Autodesk Inventor part; units mm, degrees
(part 3 of 3)
  line L2025 (60.12, -86.945) -> (55.12, -86.945)
  line L2026 (55.12, -86.945) -> (55.12, -90.12)
  line L2027 (55.12, -90.12) -> (44.88, -90.12)
  line L2028 (44.88, -90.12) -> (44.88, -86.945)
  line L2029 (44.88, -86.945) -> (35.12, -86.945)
  line L2030 (35.12, -86.945) -> (35.12, -90.12)
  line L2031 (35.12, -90.12) -> (24.88, -90.12)
  line L2032 (24.88, -90.12) -> (24.88, -86.945)
  line L2033 (24.88, -86.945) -> (15.12, -86.945)
  line L2034 (15.12, -86.945) -> (15.12, -90.12)
  line L2035 (15.12, -90.12) -> (4.88, -90.12)
  line L2036 (4.88, -90.12) -> (4.88, -86.945)
  line L2037 (4.88, -86.945) -> (-4.88, -86.945)
  line L2038 (-4.88, -86.945) -> (-4.88, -90.12)
  line L2039 (-4.88, -90.12) -> (-15.12, -90.12)
  line L2040 (-15.12, -90.12) -> (-15.12, -86.945)
  line L2041 (-15.12, -86.945) -> (-24.88, -86.945)
  line L2042 (-24.88, -86.945) -> (-24.88, -90.12)
  line L2043 (-24.88, -90.12) -> (-35.12, -90.12)
  line L2044 (-35.12, -90.12) -> (-35.12, -86.945)
  line L2045 (-35.12, -86.945) -> (-44.88, -86.945)
  line L2046 (-44.88, -86.945) -> (-44.88, -90.12)
  line L2047 (-44.88, -90.12) -> (-55.12, -90.12)
  line L2048 (-55.12, -90.12) -> (-55.12, -86.945)
  line L2049 (-55.12, -86.945) -> (-60.12, -86.945)
  line L2050 (-60.12, -86.945) -> (-60.12, -74.88)
  line L2051 (-60.12, -74.88) -> (-56.945, -74.88)
  line L2052 (-56.945, -74.88) -> (-56.945, -65.12)
  line L2053 (-56.945, -65.12) -> (-60.12, -65.12)
  line L2054 (-60.12, -65.12) -> (-60.12, -54.88)
  line L2055 (-60.12, -54.88) -> (-56.945, -54.88)
  line L2056 (-56.945, -54.88) -> (-56.945, -45.12)
  line L2057 (-56.945, -45.12) -> (-60.12, -45.12)
  line L2058 (-60.12, -45.12) -> (-60.12, -34.88)
  line L2059 (-60.12, -34.88) -> (-56.945, -34.88)
  line L2060 (-56.945, -34.88) -> (-56.945, -25.12)
  line L2061 (-56.945, -25.12) -> (-60.12, -25.12)
  line L2062 (-60.12, -25.12) -> (-60.12, -14.88)
  line L2063 (-60.12, -14.88) -> (-56.945, -14.88)
  line L2064 (145.24, 90.12) -> (155.48, 90.12)
  line L2065 (155.48, 90.12) -> (155.48, 86.945)
  line L2066 (155.48, 86.945) -> (165.24, 86.945)
  line L2067 (165.24, 86.945) -> (165.24, 90.12)
  line L2068 (165.24, 90.12) -> (175.48, 90.12)
  line L2069 (175.48, 90.12) -> (175.48, 86.945)
  line L2070 (175.48, 86.945) -> (177.305, 86.945)
  line L2071 (177.305, 86.945) -> (177.305, 75.12)
  line L2072 (177.305, 75.12) -> (180.48, 75.12)
  line L2073 (180.48, 75.12) -> (180.48, 64.88)
  line L2074 (180.48, 64.88) -> (177.305, 64.88)
  line L2075 (177.305, 64.88) -> (177.305, 55.12)
  line L2076 (177.305, 55.12) -> (180.48, 55.12)
  line L2077 (180.48, 55.12) -> (180.48, 44.88)
  line L2078 (180.48, 44.88) -> (177.305, 44.88)
  line L2079 (177.305, 44.88) -> (177.305, 35.12)
  line L2080 (177.305, 35.12) -> (180.48, 35.12)
  line L2081 (180.48, 35.12) -> (180.48, 24.88)
  line L2082 (180.48, 24.88) -> (177.305, 24.88)
  line L2083 (177.305, 24.88) -> (177.305, 15.12)
  line L2084 (177.305, 15.12) -> (180.48, 15.12)
  line L2085 (180.48, 15.12) -> (180.48, 4.88)
  line L2086 (180.48, 4.88) -> (177.305, 4.88)
  line L2087 (177.305, 4.88) -> (177.305, -4.88)
  line L2088 (177.305, -4.88) -> (180.48, -4.88)
  line L2089 (180.48, -4.88) -> (180.48, -15.12)
  line L2090 (180.48, -15.12) -> (177.305, -15.12)
  line L2091 (177.305, -15.12) -> (177.305, -24.88)
  line L2092 (177.305, -24.88) -> (180.48, -24.88)
  line L2093 (180.48, -24.88) -> (180.48, -35.12)
  line L2094 (180.48, -35.12) -> (177.305, -35.12)
  line L2095 (177.305, -35.12) -> (177.305, -44.88)
  line L2096 (177.305, -44.88) -> (180.48, -44.88)
  line L2097 (180.48, -44.88) -> (180.48, -55.12)
  line L2098 (180.48, -55.12) -> (177.305, -55.12)
  line L2099 (177.305, -55.12) -> (177.305, -64.88)
  line L2100 (177.305, -64.88) -> (180.48, -64.88)
  line L2101 (180.48, -64.88) -> (180.48, -75.12)
  line L2102 (180.48, -75.12) -> (177.305, -75.12)
  line L2103 (177.305, -75.12) -> (177.305, -86.945)
  line L2104 (177.305, -86.945) -> (175.48, -86.945)
  line L2105 (175.48, -86.945) -> (175.48, -90.12)
  line L2106 (175.48, -90.12) -> (165.24, -90.12)
  line L2107 (165.24, -90.12) -> (165.24, -86.945)
  line L2108 (165.24, -86.945) -> (155.48, -86.945)
  line L2109 (155.48, -86.945) -> (155.48, -90.12)
  line L2110 (155.48, -90.12) -> (145.24, -90.12)
  line L2111 (145.24, -90.12) -> (145.24, -86.945)
  line L2112 (145.24, -86.945) -> (135.48, -86.945)
  line L2113 (135.48, -86.945) -> (135.48, -90.12)
  line L2114 (135.48, -90.12) -> (125.24, -90.12)
  line L2115 (125.24, -90.12) -> (125.24, -86.945)
  line L2116 (125.24, -86.945) -> (115.48, -86.945)
  line L2117 (115.48, -86.945) -> (115.48, -90.12)
  line L2118 (115.48, -90.12) -> (105.24, -90.12)
  line L2119 (105.24, -90.12) -> (105.24, -86.945)
  line L2120 (105.24, -86.945) -> (95.48, -86.945)
  line L2121 (95.48, -86.945) -> (95.48, -90.12)
  line L2122 (95.48, -90.12) -> (85.24, -90.12)
  line L2123 (85.24, -90.12) -> (85.24, -86.945)
  line L2124 (85.24, -86.945) -> (75.48, -86.945)
  line L2125 (75.48, -86.945) -> (75.48, -90.12)
  line L2126 (75.48, -90.12) -> (65.24, -90.12)
  line L2127 (65.24, -90.12) -> (65.24, -86.945)
  line L2128 (65.24, -86.945) -> (63.415, -86.945)
  line L2129 (63.415, -86.945) -> (63.415, -75.12)
  line L2130 (63.415, -75.12) -> (60.24, -75.12)
  line L2131 (60.24, -75.12) -> (60.24, -64.88)
  line L2132 (60.24, -64.88) -> (63.415, -64.88)
  line L2133 (63.415, -64.88) -> (63.415, -55.12)
  line L2134 (63.415, -55.12) -> (60.24, -55.12)
  line L2135 (60.24, -55.12) -> (60.24, -44.88)
  line L2136 (60.24, -44.88) -> (63.415, -44.88)
  line L2137 (63.415, -44.88) -> (63.415, -35.12)
  line L2138 (63.415, -35.12) -> (60.24, -35.12)
  line L2139 (60.24, -35.12) -> (60.24, -24.88)
  line L2140 (60.24, -24.88) -> (63.415, -24.88)
  line L2141 (63.415, -24.88) -> (63.415, -15.12)
  line L2142 (63.415, -15.12) -> (60.24, -15.12)
  line L2143 (60.24, -15.12) -> (60.24, -4.88)
  line L2144 (60.24, -4.88) -> (63.415, -4.88)
  line L2145 (63.415, -4.88) -> (63.415, 4.88)
  line L2146 (63.415, 4.88) -> (60.24, 4.88)
  line L2147 (60.24, 4.88) -> (60.24, 15.12)
  line L2148 (60.24, 15.12) -> (63.415, 15.12)
  line L2149 (63.415, 15.12) -> (63.415, 24.88)
  line L2150 (63.415, 24.88) -> (60.24, 24.88)
  line L2151 (60.24, 24.88) -> (60.24, 35.12)
  line L2152 (60.24, 35.12) -> (63.415, 35.12)
  line L2153 (63.415, 35.12) -> (63.415, 44.88)
  line L2154 (63.415, 44.88) -> (60.24, 44.88)
  line L2155 (60.24, 44.88) -> (60.24, 55.12)
  line L2156 (60.24, 55.12) -> (63.415, 55.12)
  line L2157 (63.415, 55.12) -> (63.415, 64.88)
  line L2158 (63.415, 64.88) -> (60.24, 64.88)
  line L2159 (60.24, 64.88) -> (60.24, 75.12)
  line L2160 (60.24, 75.12) -> (63.415, 75.12)
  line L2161 (63.415, 75.12) -> (63.415, 86.945)
  line L2162 (63.415, 86.945) -> (65.24, 86.945)
  line L2163 (65.24, 86.945) -> (65.24, 90.12)
  line L2164 (65.24, 90.12) -> (75.48, 90.12)
  line L2165 (75.48, 90.12) -> (75.48, 86.945)
  line L2166 (75.48, 86.945) -> (85.24, 86.945)
  line L2167 (85.24, 86.945) -> (85.24, 90.12)
  line L2168 (85.24, 90.12) -> (95.48, 90.12)
  line L2169 (95.48, 90.12) -> (95.48, 86.945)
  line L2170 (95.48, 86.945) -> (105.24, 86.945)
  line L2171 (105.24, 86.945) -> (105.24, 90.12)
  line L2172 (105.24, 90.12) -> (115.48, 90.12)
  line L2173 (115.48, 90.12) -> (115.48, 86.945)
  line L2174 (115.48, 86.945) -> (125.24, 86.945)
  line L2175 (125.24, 86.945) -> (125.24, 90.12)
  line L2176 (125.24, 90.12) -> (135.48, 90.12)
  line L2177 (135.48, 90.12) -> (135.48, 86.945)
  line L2178 (135.48, 86.945) -> (145.24, 86.945)
  line L2179 (145.24, 86.945) -> (145.24, 90.12)
  line L2180 (165.48, 14.88) -> (165.48, -14.88)
  line L2181 (165.48, -14.88) -> (175.24, -14.88)
  line L2182 (175.24, -14.88) -> (175.24, 14.88)
  line L2183 (175.24, 14.88) -> (165.48, 14.88)
  line L2184 (75.24, 14.88) -> (65.48, 14.88)
  line L2185 (65.48, 14.88) -> (65.48, -14.88)
  line L2186 (65.48, -14.88) -> (75.24, -14.88)
  line L2187 (75.24, -14.88) -> (75.24, 14.88)
  circle A54 centre (177.185, 50) radius 1.58
  circle A55 centre (177.185, -50) radius 1.58
  circle A56 centre (22.9972, 27.4451) radius 2.88
  line L2188 (43.695, -13.215) -> (40.125, -13.215)
  line L2189 (40.125, -13.215) -> (40.125, -2.025)
  line L2190 (40.125, -2.025) -> (43.695, -2.025)
  line L2191 (43.695, -2.025) -> (43.695, -13.215)
  circle A57 centre (45.72, 0) radius 0.958
  circle A58 centre (45.72, -15.24) radius 0.958
  circle A59 centre (38.1, -15.24) radius 0.958
  circle A60 centre (38.1, 0) radius 0.958
  circle A61 centre (22.9972, -27.4451) radius 2.88
  circle A62 centre (-15, 8.175) radius 11.12
  circle A63 centre (-22.9972, 54) radius 2.88
  circle A64 centre (-22.9972, -54) radius 2.88
  circle A65 centre (17.276, -59.1479) radius 0.958
  circle A66 centre (52.276, -59.1479) radius 0.958
  circle A67 centre (63.535, -50) radius 1.58
  circle A68 centre (63.535, 50) radius 1.58
  line L2192 (404.895, -13.335) -> (401.085, -13.335) projected
  line L2193 (401.085, -13.335) -> (401.085, -1.905) projected
  line L2194 (401.085, -1.905) -> (404.895, -1.905) projected
  line L2195 (404.895, -1.905) -> (404.895, -13.335) projected
  circle A69 centre (399.18, -15.24) radius 1.078 projected
  circle A70 centre (406.8, 0) radius 1.078 projected
  circle A71 centre (406.8, -15.24) radius 1.078 projected
  circle A72 centre (399.18, 0) radius 1.078 projected
  line L2196 (415.905, -48.5) -> (417.905, -48.5) projected
  line L2197 (417.905, -48.5) -> (417.905, -45) projected
  line L2198 (417.905, -45) -> (421.08, -45) projected
  line L2199 (421.08, -45) -> (421.08, -35) projected
  line L2200 (421.08, -35) -> (417.905, -35) projected
  line L2201 (417.905, -35) -> (417.905, -25) projected
  line L2202 (417.905, -25) -> (421.08, -25) projected
  line L2203 (421.08, -25) -> (421.08, -15) projected
  line L2204 (421.08, -15) -> (417.905, -15) projected
  line L2205 (417.905, -15) -> (417.905, -5) projected
  line L2206 (417.905, -5) -> (421.08, -5) projected
  line L2207 (421.08, -5) -> (421.08, 5) projected
  line L2208 (421.08, 5) -> (417.905, 5) projected
  line L2209 (417.905, 5) -> (417.905, 15) projected
  line L2210 (417.905, 15) -> (421.08, 15) projected
  line L2211 (421.08, 15) -> (421.08, 25) projected
  line L2212 (421.08, 25) -> (417.905, 25) projected
  line L2213 (417.905, 25) -> (417.905, 35) projected
  line L2214 (417.905, 35) -> (421.08, 35) projected
  line L2215 (421.08, 35) -> (421.08, 45) projected
  line L2216 (421.08, 45) -> (417.905, 45) projected
  line L2217 (417.905, 45) -> (417.905, 48.5) projected
  line L2218 (417.905, 48.5) -> (415.905, 48.5) projected
  line L2219 (415.905, 48.5) -> (415.905, 47.25) projected
  line L2220 (415.905, 47.25) -> (413.405, 47.25) projected
  line L2221 (413.405, 47.25) -> (413.405, 48.5) projected
  line L2222 (413.405, 48.5) -> (407.08, 48.5) projected
  line L2223 (407.08, 48.5) -> (407.08, 51.5) projected
  line L2224 (407.08, 51.5) -> (413.405, 51.5) projected
  line L2225 (413.405, 51.5) -> (413.405, 52.75) projected
  line L2226 (413.405, 52.75) -> (415.905, 52.75) projected
  line L2227 (415.905, 52.75) -> (415.905, 51.5) projected
  line L2228 (415.905, 51.5) -> (417.905, 51.5) projected
  line L2229 (417.905, 51.5) -> (417.905, 55) projected
  line L2230 (417.905, 55) -> (421.08, 55) projected
  line L2231 (421.08, 55) -> (421.08, 65) projected
  line L2232 (421.08, 65) -> (417.905, 65) projected
  line L2233 (417.905, 65) -> (417.905, 75) projected
  line L2234 (417.905, 75) -> (421.08, 75) projected
  line L2235 (421.08, 75) -> (421.08, 86.825) projected
  line L2236 (416.08, 86.825) -> (421.08, 86.825) projected
  line L2237 (416.08, 90) -> (416.08, 86.825) projected
  line L2238 (406.08, 90) -> (416.08, 90) projected
  line L2239 (406.08, 86.825) -> (406.08, 90) projected
  line L2240 (406.08, 86.825) -> (396.08, 86.825) projected
  line L2241 (396.08, 90) -> (396.08, 86.825) projected
  line L2242 (386.08, 90) -> (396.08, 90) projected
  line L2243 (386.08, 86.825) -> (386.08, 90) projected
  line L2244 (386.08, 86.825) -> (376.08, 86.825) projected
  line L2245 (376.08, 90) -> (376.08, 86.825) projected
  line L2246 (366.08, 90) -> (376.08, 90) projected
  line L2247 (366.08, 86.825) -> (366.08, 90) projected
  line L2248 (366.08, 86.825) -> (356.08, 86.825) projected
  line L2249 (356.08, 90) -> (356.08, 86.825) projected
  line L2250 (346.08, 90) -> (356.08, 90) projected
  line L2251 (346.08, 86.825) -> (346.08, 90) projected
  line L2252 (346.08, 86.825) -> (336.08, 86.825) projected
  line L2253 (336.08, 90) -> (336.08, 86.825) projected
  line L2254 (326.08, 90) -> (336.08, 90) projected
  line L2255 (326.08, 86.825) -> (326.08, 90) projected
  line L2256 (326.08, 86.825) -> (316.08, 86.825) projected
  line L2257 (316.08, 90) -> (316.08, 86.825) projected
  line L2258 (306.08, 90) -> (316.08, 90) projected
  line L2259 (306.08, 86.825) -> (306.08, 90) projected
  line L2260 (306.08, 86.825) -> (301.08, 86.825) projected
  line L2261 (301.08, 75) -> (301.08, 86.825) projected
  line L2262 (304.255, 75) -> (301.08, 75) projected
  line L2263 (304.255, 75) -> (304.255, 65) projected
  line L2264 (301.08, 65) -> (304.255, 65) projected
  line L2265 (301.08, 55) -> (301.08, 65) projected
  line L2266 (304.255, 55) -> (301.08, 55) projected
  line L2267 (304.255, 55) -> (304.255, 45) projected
  line L2268 (301.08, 45) -> (304.255, 45) projected
  line L2269 (301.08, 35) -> (301.08, 45) projected
  line L2270 (304.255, 35) -> (301.08, 35) projected
  line L2271 (304.255, 35) -> (304.255, 25) projected
  line L2272 (301.08, 25) -> (304.255, 25) projected
  line L2273 (301.08, 15) -> (301.08, 25) projected
  line L2274 (304.255, 15) -> (301.08, 15) projected
  line L2275 (304.255, 15) -> (304.255, 5) projected
  line L2276 (301.08, 5) -> (304.255, 5) projected
  line L2277 (301.08, -5) -> (301.08, 5) projected
  line L2278 (304.255, -5) -> (301.08, -5) projected
  line L2279 (304.255, -5) -> (304.255, -15) projected
  line L2280 (301.08, -15) -> (304.255, -15) projected
  line L2281 (301.08, -25) -> (301.08, -15) projected
  line L2282 (304.255, -25) -> (301.08, -25) projected
  line L2283 (304.255, -25) -> (304.255, -35) projected
  line L2284 (301.08, -35) -> (304.255, -35) projected
  line L2285 (301.08, -45) -> (301.08, -35) projected
  line L2286 (304.255, -45) -> (301.08, -45) projected
  line L2287 (304.255, -45) -> (304.255, -55) projected
  line L2288 (301.08, -55) -> (304.255, -55) projected
  line L2289 (301.08, -65) -> (301.08, -55) projected
  line L2290 (304.255, -65) -> (301.08, -65) projected
  line L2291 (304.255, -65) -> (304.255, -75) projected
  line L2292 (301.08, -75) -> (304.255, -75) projected
  line L2293 (301.08, -75) -> (301.08, -86.825) projected
  line L2294 (301.08, -86.825) -> (306.08, -86.825) projected
  line L2295 (306.08, -86.825) -> (306.08, -90) projected
  line L2296 (306.08, -90) -> (316.08, -90) projected
  line L2297 (316.08, -90) -> (316.08, -86.825) projected
  line L2298 (316.08, -86.825) -> (326.08, -86.825) projected
  line L2299 (326.08, -86.825) -> (326.08, -90) projected
  line L2300 (326.08, -90) -> (336.08, -90) projected
  line L2301 (336.08, -90) -> (336.08, -86.825) projected
  line L2302 (336.08, -86.825) -> (346.08, -86.825) projected
  line L2303 (346.08, -86.825) -> (346.08, -90) projected
  line L2304 (346.08, -90) -> (356.08, -90) projected
  line L2305 (356.08, -90) -> (356.08, -86.825) projected
  line L2306 (356.08, -86.825) -> (366.08, -86.825) projected
  line L2307 (366.08, -86.825) -> (366.08, -90) projected
  line L2308 (366.08, -90) -> (376.08, -90) projected
  line L2309 (376.08, -90) -> (376.08, -86.825) projected
  line L2310 (376.08, -86.825) -> (386.08, -86.825) projected
  line L2311 (386.08, -86.825) -> (386.08, -90) projected
  line L2312 (386.08, -90) -> (396.08, -90) projected
  line L2313 (396.08, -90) -> (396.08, -86.825) projected
  line L2314 (396.08, -86.825) -> (406.08, -86.825) projected
  line L2315 (406.08, -86.825) -> (406.08, -90) projected
  line L2316 (406.08, -90) -> (416.08, -90) projected
  line L2317 (416.08, -90) -> (416.08, -86.825) projected
  line L2318 (416.08, -86.825) -> (421.08, -86.825) projected
  line L2319 (421.08, -86.825) -> (421.08, -75) projected
  line L2320 (421.08, -75) -> (417.905, -75) projected
  line L2321 (417.905, -75) -> (417.905, -65) projected
  line L2322 (417.905, -65) -> (421.08, -65) projected
  line L2323 (421.08, -65) -> (421.08, -55) projected
  line L2324 (421.08, -55) -> (417.905, -55) projected
  line L2325 (417.905, -55) -> (417.905, -51.5) projected
  line L2326 (417.905, -51.5) -> (415.905, -51.5) projected
  line L2327 (415.905, -51.5) -> (415.905, -52.75) projected
  line L2328 (415.905, -52.75) -> (413.405, -52.75) projected
  line L2329 (413.405, -52.75) -> (413.405, -51.5) projected
  line L2330 (413.405, -51.5) -> (407.08, -51.5) projected
  line L2331 (407.08, -51.5) -> (407.08, -48.5) projected
  line L2332 (407.08, -48.5) -> (413.405, -48.5) projected
  line L2333 (413.405, -48.5) -> (413.405, -47.25) projected
  line L2334 (413.405, -47.25) -> (415.905, -47.25) projected
  line L2335 (415.905, -47.25) -> (415.905, -48.5) projected
  circle A73 centre (384.0772, -27.4451) radius 3 projected
  circle A74 centre (338.0828, 54) radius 3 projected
  circle A75 centre (384.0772, 27.4451) radius 3 projected
  circle A76 centre (338.0828, -54) radius 3 projected
  circle A77 centre (346.08, 8.175) radius 11 projected
  point P0 (0, 0)
  dimension "d0" = 0.12
  dimension "d1" = 0.12
  dimension "d2" = 0.12
  dimension "d3" = 0.12
  dimension "d4" = 0.12
  dimension "d5" = 0.12
  dimension "d6" = 0.12
  dimension "d7" = 0.12
  dimension "d8" = 0.12
  dimension "d9" = 0.12
  dimension "d10" = 0.12
  dimension "d11" = 0.12
  dimension "d12" = 0.12
  dimension "d13" = 0.12
  dimension "d14" = 0.12
  dimension "d15" = 0.12
  dimension "d16" = 0.12
  dimension "d17" = 0.12
  dimension "d18" = 0.12
  dimension "d19" = 0.12
  dimension "d20" = 0.12
  dimension "d21" = 0.12
  dimension "d22" = 0.12
  dimension "d23" = 0.12
  dimension "d24" = 0.12
  dimension "d25" = 0.12
  dimension "d26" = 0.12
  dimension "d27" = 0.12
  dimension "d28" = 0.12
  dimension "d29" = 0.12
  dimension "d30" = 0.12
  dimension "d31" = 0.12
  dimension "d32" = 0.12
  dimension "d33" = 0.12
  dimension "d34" = 0.12
  dimension "d35" = 0.12
  dimension "d36" = 0.12
  dimension "d37" = 0.12
  dimension "d38" = 0.12
  constraints: 1904 end point, 25 centre point, 938 other
  measures "d0" distance between parallel lines of L995 L1096
  measures "d1" radial gap between concentric circles of A27 A35
  measures "d2" radial gap between concentric circles of A29 A36
  measures "d3" distance between parallel lines of L955 L1239
  measures "d4" radial gap between concentric circles of A28 A37
  measures "d5" radial gap between concentric circles of A26 A38
  measures "d6" radial gap between concentric circles of A32 A39
  measures "d7" radial gap between concentric circles of A30 A40
  measures "d8" radial gap between concentric circles of A24 A41
  measures "d9" radial gap between concentric circles of A25 A42
  measures "d10" radial gap between concentric circles of A31 A43
  measures "d11" radial gap between concentric circles of A34 A44
  measures "d12" distance between parallel lines of L685 L1384
  measures "d13" distance between parallel lines of L575 L1388
  measures "d14" distance between parallel lines of L876 L1504
  measures "d15" distance between parallel lines of L948 L1620
  measures "d16" distance between parallel lines of L567 L1723
  measures "d17" distance between parallel lines of L337 L1724
  measures "d18" distance between parallel lines of L233 L1824
  measures "d19" distance between parallel lines of L87 L1924
  measures "d20" distance between parallel lines of L359 L2064
  measures "d21" distance between parallel lines of L344 L2180
  measures "d22" distance between parallel lines of L349 L2184
  measures "d23" radial gap between concentric circles of A12 A54
  measures "d24" radial gap between concentric circles of A11 A55
  measures "d25" radial gap between concentric circles of A8 A56
  measures "d26" distance between parallel lines of L3 L2191
  measures "d27" radial gap between concentric circles of A3 A57
  measures "d28" radial gap between concentric circles of A4 A58
  measures "d29" radial gap between concentric circles of A2 A59
  measures "d30" radial gap between concentric circles of A5 A60
  measures "d31" radial gap between concentric circles of A6 A61
  measures "d32" radial gap between concentric circles of A10 A62
  measures "d33" radial gap between concentric circles of A7 A63
  measures "d34" radial gap between concentric circles of A9 A64
  measures "d35" radial gap between concentric circles of A1 A65
  measures "d36" radial gap between concentric circles of A0 A66
  measures "d37" radial gap between concentric circles of A13 A67
  measures "d38" radial gap between concentric circles of A14 A68
extrude "Extrusion1" add sketch "Sketch1" along normal blind 3.175 contours A0 | A1 | L0 L1 L2 L3 | A2 | A3 | A4 | A5 | L143 L142 L141 L140 L139 L138 L137 L136 L135 L134 L133 L132 L131 L130 L129 L128 L127 L126 L125 L124 L123 L122 L121 L120 L119 L118 L117 L116 L115 L114 L113 L112 L111 L110 L109 L108 L107 L106 L105 L104 L103 L102 L101 L100 L99 L98 L97 L96 L95 L94 L93 L92 L91 L90 L89 L88 L87 L86 L85 L84 L83 L82 L81 L80 L79 L78 L77 L76 L75 L74 L73 L72 L71 L70 L69 L68 L67 L66 L65 L64 L63 L62 L61 L60 L59 L58 L57 L56 L55 L54 L53 L52 L51 L50 L49 L48 L47 L46 L45 L44 L43 L42 L41 L40 L39 L38 L37 L36 L35 L34 L33 L32 L31 L30 L29 L28 L27 L26 L25 L24 L23 L22 L21 L20 L19 L18 L17 L16 L15 L14 L13 L12 L11 L10 L9 L8 L7 L6 L5 L4 | A6 | A7 | A8 | A9 | L243 L242 L241 L240 L239 L238 L237 L236 L235 L234 L233 L232 L231 L230 L229 L228 L227 L226 L225 L224 L223 L222 L221 L220 L219 L218 L217 L216 L215 L214 L213 L212 L211 L210 L209 L208 L207 L206 L205 L204 L203 L202 L201 L200 L199 L198 L197 L196 L195 L194 L193 L192 L191 L190 L189 L188 L187 L186 L185 L184 L183 L182 L181 L180 L179 L178 L177 L176 L175 L174 L173 L172 L171 L170 L169 L168 L167 L166 L165 L164 L163 L162 L161 L160 L159 L158 L157 L156 L155 L154 L153 L152 L151 L150 L149 L148 L147 L146 L145 L144 | L343 L342 L341 L340 L339 L338 L337 L336 L335 L334 L333 L332 L331 L330 L329 L328 L327 L326 L325 L324 L323 L322 L321 L320 L319 L318 L317 L316 L315 L314 L313 L312 L311 L310 L309 L308 L307 L306 L305 L304 L303 L302 L301 L300 L299 L298 L297 L296 L295 L294 L293 L292 L291 L290 L289 L288 L287 L286 L285 L284 L283 L282 L281 L280 L279 L278 L277 L276 L275 L274 L273 L272 L271 L270 L269 L268 L267 L266 L265 L264 L263 L262 L261 L260 L259 L258 L257 L256 L255 L254 L253 L252 L251 L250 L249 L248 L247 L246 L245 L244 | L344 L345 L346 L347 | L348 L349 L350 L351 | A11 | A12 | A13 | A14 | L467 L466 L465 L464 L463 L462 L461 L460 L459 L458 L457 L456 L455 L454 L453 L452 L451 L450 L449 L448 L447 L446 L445 L444 L443 L442 L441 L440 L439 L438 L437 L436 L435 L434 L433 L432 L431 L430 L429 L428 L427 L426 L425 L424 L423 L422 L421 L420 L419 L418 L417 L416 L415 L414 L413 L412 L411 L410 L409 L408 L407 L406 L405 L404 L403 L402 L401 L400 L399 L398 L397 L396 L395 L394 L393 L392 L391 L390 L389 L388 L387 L386 L385 L384 L383 L382 L381 L380 L379 L378 L377 L376 L375 L374 L373 L372 L371 L370 L369 L368 L367 L366 L365 L364 L363 L362 L361 L360 L359 L358 L357 L356 L355 L354 L353 L352 | L567 L566 L565 L564 L563 L562 L561 L560 L559 L558 L557 L556 L555 L554 L553 L552 L551 L550 L549 L548 L547 L546 L545 L544 L543 L542 L541 L540 L539 L538 L537 L536 L535 L534 L533 L532 L531 L530 L529 L528 L527 L526 L525 L524 L523 L522 L521 L520 L519 L518 L517 L516 L515 L514 L513 L512 L511 L510 L509 L508 L507 L506 L505 L504 L503 L502 L501 L500 L499 L498 L497 L496 L495 L494 L493 L492 L491 L490 L489 L488 L487 L486 L485 L484 L483 L482 L481 L480 L479 L478 L477 L476 L475 L474 L473 L472 L471 L470 L469 L468 | L683 L682 L681 L680 L679 L678 L677 L676 L675 L674 L673 L672 L671 L670 L669 L668 L667 L666 L665 L664 L663 L662 L661 L660 L659 L658 L657 L656 L655 L654 L653 L652 L651 L650 L649 L648 L647 L646 L645 L644 L643 L642 L641 L640 L639 L638 L637 L636 L635 L634 L633 L632 L631 L630 L629 L628 L627 L626 L625 L624 L623 L622 L621 L620 L619 L618 L617 L616 L615 L614 L613 L612 L611 L610 L609 L608 L607 L606 L605 L604 L603 L602 L601 L600 L599 L598 L597 L596 L595 L594 L593 L592 L591 L590 L589 L588 L587 L586 L585 L584 L583 L582 L581 L580 L579 L578 L577 L576 L575 L574 L573 L572 L571 L570 L569 L568 | L684 L685 L686 L687 | L947 L946 L945 L944 L943 L942 L941 L940 L939 L938 L937 L936 L935 L934 L933 L932 L931 L930 L929 L928 L927 L926 L925 L924 L923 L922 L921 L920 L919 L918 L917 L916 L915 L914 L913 L912 L911 L910 L909 L908 L907 L906 L905 L904 L903 L902 L901 L900 L899 L898 L897 L896 L895 L894 L893 L892 L891 L890 L889 L888 L887 L886 L885 L884 L883 L882 L881 L880 L879 L878 L877 L876 L875 L874 L873 L872 L871 L870 L869 L868 L867 L866 L865 L864 L863 L862 L861 L860 L859 L858 L857 L856 L855 L854 L853 L852 L851 L850 L849 L848 L847 L846 L845 L844 L843 L842 L841 L840 L839 L838 L837 L836 L835 L834 L833 L832 | L948 L949 L950 L951 | A24 | A25 | L952 L953 L954 L955 | A27 | A28 | A29 | L1095 L1094 L1093 L1092 L1091 L1090 L1089 L1088 L1087 L1086 L1085 L1084 L1083 L1082 L1081 L1080 L1079 L1078 L1077 L1076 L1075 L1074 L1073 L1072 L1071 L1070 L1069 L1068 L1067 L1066 L1065 L1064 L1063 L1062 L1061 L1060 L1059 L1058 L1057 L1056 L1055 L1054 L1053 L1052 L1051 L1050 L1049 L1048 L1047 L1046 L1045 L1044 L1043 L1042 L1041 L1040 L1039 L1038 L1037 L1036 L1035 L1034 L1033 L1032 L1031 L1030 L1029 L1028 L1027 L1026 L1025 L1024 L1023 L1022 L1021 L1020 L1019 L1018 L1017 L1016 L1015 L1014 L1013 L1012 L1011 L1010 L1009 L1008 L1007 L1006 L1005 L1004 L1003 L1002 L1001 L1000 L999 L998 L997 L996 L995 L994 L993 L992 L991 L990 L989 L988 L987 L986 L985 L984 L983 L982 L981 L980 L979 L978 L977 L976 L975 L974 L973 L972 L971 L970 L969 L968 L967 L966 L965 L964 L963 L962 L961 L960 L959 L958 L957 L956 | A30 | A31 | A32 | A34 | L1096 L1097 L1098 L1099 L1100 L1101 L1102 L1103 L1104 L1105 L1106 L1107 L1108 L1109 L1110 L1111 L1112 L1113 L1114 L1115 L1116 L1117 L1118 L1119 L1120 L1121 L1122 L1123 L1124 L1125 L1126 L1127 L1128 L1129 L1130 L1131 L1132 L1133 L1134 L1135 L1136 L1137 L1138 L1139 L1140 L1141 L1142 L1143 L1144 L1145 L1146 L1147 L1148 L1149 L1150 L1151 L1152 L1153 L1154 L1155 L1156 L1157 L1158 L1159 L1160 L1161 L1162 L1163 L1164 L1165 L1166 L1167 L1168 L1169 L1170 L1171 L1172 L1173 L1174 L1175 L1176 L1177 L1178 L1179 L1180 L1181 L1182 L1183 L1184 L1185 L1186 L1187 L1188 L1189 L1190 L1191 L1192 L1193 L1194 L1195 L1196 L1197 L1198 L1199 L1200 L1201 L1202 L1203 L1204 L1205 L1206 L1207 L1208 L1209 L1210 L1211 L1212 L1213 L1214 L1215 L1216 L1217 L1218 L1219 L1220 L1221 L1222 L1223 L1224 L1225 L1226 L1227 L1228 L1229 L1230 L1231 L1232 L1233 L1234 L1235 | A38 | L1388 L1389 L1390 L1391 L1392 L1393 L1394 L1395 L1396 L1397 L1398 L1399 L1400 L1401 L1402 L1403 L1404 L1405 L1406 L1407 L1408 L1409 L1410 L1411 L1412 L1413 L1414 L1415 L1416 L1417 L1418 L1419 L1420 L1421 L1422 L1423 L1424 L1425 L1426 L1427 L1428 L1429 L1430 L1431 L1432 L1433 L1434 L1435 L1436 L1437 L1438 L1439 L1440 L1441 L1442 L1443 L1444 L1445 L1446 L1447 L1448 L1449 L1450 L1451 L1452 L1453 L1454 L1455 L1456 L1457 L1458 L1459 L1460 L1461 L1462 L1463 L1464 L1465 L1466 L1467 L1468 L1469 L1470 L1471 L1472 L1473 L1474 L1475 L1476 L1477 L1478 L1479 L1480 L1481 L1482 L1483 L1484 L1485 L1486 L1487 L1488 L1489 L1490 L1491 L1492 L1493 L1494 L1495 L1496 L1497 L1498 L1499 L1500 L1501 L1502 L1503 | L1504 L1505 L1506 L1507 L1508 L1509 L1510 L1511 L1512 L1513 L1514 L1515 L1516 L1517 L1518 L1519 L1520 L1521 L1522 L1523 L1524 L1525 L1526 L1527 L1528 L1529 L1530 L1531 L1532 L1533 L1534 L1535 L1536 L1537 L1538 L1539 L1540 L1541 L1542 L1543 L1544 L1545 L1546 L1547 L1548 L1549 L1550 L1551 L1552 L1553 L1554 L1555 L1556 L1557 L1558 L1559 L1560 L1561 L1562 L1563 L1564 L1565 L1566 L1567 L1568 L1569 L1570 L1571 L1572 L1573 L1574 L1575 L1576 L1577 L1578 L1579 L1580 L1581 L1582 L1583 L1584 L1585 L1586 L1587 L1588 L1589 L1590 L1591 L1592 L1593 L1594 L1595 L1596 L1597 L1598 L1599 L1600 L1601 L1602 L1603 L1604 L1605 L1606 L1607 L1608 L1609 L1610 L1611 L1612 L1613 L1614 L1615 L1616 L1617 L1618 L1619 | L1723 L1722 L1721 L1720 L1719 L1718 L1717 L1716 L1715 L1714 L1713 L1712 L1711 L1710 L1709 L1708 L1707 L1706 L1705 L1704 L1703 L1702 L1701 L1700 L1699 L1698 L1697 L1696 L1695 L1694 L1693 L1692 L1691 L1690 L1689 L1688 L1687 L1686 L1685 L1684 L1683 L1682 L1681 L1680 L1679 L1678 L1677 L1676 L1675 L1674 L1673 L1672 L1671 L1670 L1669 L1668 L1667 L1666 L1665 L1664 L1663 L1662 L1661 L1660 L1659 L1658 L1657 L1656 L1655 L1654 L1653 L1652 L1651 L1650 L1649 L1648 L1647 L1646 L1645 L1644 L1643 L1642 L1641 L1640 L1639 L1638 L1637 L1636 L1635 L1634 L1633 L1632 L1631 L1630 L1629 L1628 L1627 L1626 L1625 L1624 | L1724 L1725 L1726 L1727 L1728 L1729 L1730 L1731 L1732 L1733 L1734 L1735 L1736 L1737 L1738 L1739 L1740 L1741 L1742 L1743 L1744 L1745 L1746 L1747 L1748 L1749 L1750 L1751 L1752 L1753 L1754 L1755 L1756 L1757 L1758 L1759 L1760 L1761 L1762 L1763 L1764 L1765 L1766 L1767 L1768 L1769 L1770 L1771 L1772 L1773 L1774 L1775 L1776 L1777 L1778 L1779 L1780 L1781 L1782 L1783 L1784 L1785 L1786 L1787 L1788 L1789 L1790 L1791 L1792 L1793 L1794 L1795 L1796 L1797 L1798 L1799 L1800 L1801 L1802 L1803 L1804 L1805 L1806 L1807 L1808 L1809 L1810 L1811 L1812 L1813 L1814 L1815 L1816 L1817 L1818 L1819 L1820 L1821 L1822 L1823 | L1824 L1825 L1826 L1827 L1828 L1829 L1830 L1831 L1832 L1833 L1834 L1835 L1836 L1837 L1838 L1839 L1840 L1841 L1842 L1843 L1844 L1845 L1846 L1847 L1848 L1849 L1850 L1851 L1852 L1853 L1854 L1855 L1856 L1857 L1858 L1859 L1860 L1861 L1862 L1863 L1864 L1865 L1866 L1867 L1868 L1869 L1870 L1871 L1872 L1873 L1874 L1875 L1876 L1877 L1878 L1879 L1880 L1881 L1882 L1883 L1884 L1885 L1886 L1887 L1888 L1889 L1890 L1891 L1892 L1893 L1894 L1895 L1896 L1897 L1898 L1899 L1900 L1901 L1902 L1903 L1904 L1905 L1906 L1907 L1908 L1909 L1910 L1911 L1912 L1913 L1914 L1915 L1916 L1917 L1918 L1919 L1920 L1921 L1922 L1923 | L1924 L1925 L1926 L1927 L1928 L1929 L1930 L1931 L1932 L1933 L1934 L1935 L1936 L1937 L1938 L1939 L1940 L1941 L1942 L1943 L1944 L1945 L1946 L1947 L1948 L1949 L1950 L1951 L1952 L1953 L1954 L1955 L1956 L1957 L1958 L1959 L1960 L1961 L1962 L1963 L1964 L1965 L1966 L1967 L1968 L1969 L1970 L1971 L1972 L1973 L1974 L1975 L1976 L1977 L1978 L1979 L1980 L1981 L1982 L1983 L1984 L1985 L1986 L1987 L1988 L1989 L1990 L1991 L1992 L1993 L1994 L1995 L1996 L1997 L1998 L1999 L2000 L2001 L2002 L2003 L2004 L2005 L2006 L2007 L2008 L2009 L2010 L2011 L2012 L2013 L2014 L2015 L2016 L2017 L2018 L2019 L2020 L2021 L2022 L2023 L2024 L2025 L2026 L2027 L2028 L2029 L2030 L2031 L2032 L2033 L2034 L2035 L2036 L2037 L2038 L2039 L2040 L2041 L2042 L2043 L2044 L2045 L2046 L2047 L2048 L2049 L2050 L2051 L2052 L2053 L2054 L2055 L2056 L2057 L2058 L2059 L2060 L2061 L2062 L2063 | L2064 L2065 L2066 L2067 L2068 L2069 L2070 L2071 L2072 L2073 L2074 L2075 L2076 L2077 L2078 L2079 L2080 L2081 L2082 L2083 L2084 L2085 L2086 L2087 L2088 L2089 L2090 L2091 L2092 L2093 L2094 L2095 L2096 L2097 L2098 L2099 L2100 L2101 L2102 L2103 L2104 L2105 L2106 L2107 L2108 L2109 L2110 L2111 L2112 L2113 L2114 L2115 L2116 L2117 L2118 L2119 L2120 L2121 L2122 L2123 L2124 L2125 L2126 L2127 L2128 L2129 L2130 L2131 L2132 L2133 L2134 L2135 L2136 L2137 L2138 L2139 L2140 L2141 L2142 L2143 L2144 L2145 L2146 L2147 L2148 L2149 L2150 L2151 L2152 L2153 L2154 L2155 L2156 L2157 L2158 L2159 L2160 L2161 L2162 L2163 L2164 L2165 L2166 L2167 L2168 L2169 L2170 L2171 L2172 L2173 L2174 L2175 L2176 L2177 L2178 L2179 | A62
ref_plane "Work Plane2" through (361.08, 0, 0) normal (0, 0, 1) x (1, 0, 0)
sketch "Sketch3" plane through (361.08, 0, 0) normal (0, 0, 1) x (1, 0, 0)
  line L0 (43.815, -13.335) -> (40.005, -13.335) projected
  line L1 (40.005, -13.335) -> (40.005, -1.905) projected
  line L2 (40.005, -1.905) -> (43.815, -1.905) projected
  line L3 (43.815, -1.905) -> (43.815, -13.335) projected
  circle A0 centre (38.1, -15.24) radius 1.078 projected
  circle A1 centre (45.72, 0) radius 1.078 projected
  circle A2 centre (45.72, -15.24) radius 1.078 projected
  circle A3 centre (38.1, 0) radius 1.078 projected
  line L4 (54.825, -48.5) -> (56.825, -48.5) projected
  line L5 (56.825, -48.5) -> (56.825, -45) projected
  line L6 (56.825, -45) -> (60, -45) projected
  line L7 (60, -45) -> (60, -35) projected
  line L8 (60, -35) -> (56.825, -35) projected
  line L9 (56.825, -35) -> (56.825, -25) projected
  line L10 (56.825, -25) -> (60, -25) projected
  line L11 (60, -25) -> (60, -15) projected
  line L12 (60, -15) -> (56.825, -15) projected
  line L13 (56.825, -15) -> (56.825, -5) projected
  line L14 (56.825, -5) -> (60, -5) projected
  line L15 (60, -5) -> (60, 5) projected
  line L16 (60, 5) -> (56.825, 5) projected
  line L17 (56.825, 5) -> (56.825, 15) projected
  line L18 (56.825, 15) -> (60, 15) projected
  line L19 (60, 15) -> (60, 25) projected
  line L20 (60, 25) -> (56.825, 25) projected
  line L21 (56.825, 25) -> (56.825, 35) projected
  line L22 (56.825, 35) -> (60, 35) projected
  line L23 (60, 35) -> (60, 45) projected
  line L24 (60, 45) -> (56.825, 45) projected
  line L25 (56.825, 45) -> (56.825, 48.5) projected
  line L26 (56.825, 48.5) -> (54.825, 48.5) projected
  line L27 (54.825, 48.5) -> (54.825, 47.25) projected
  line L28 (54.825, 47.25) -> (52.325, 47.25) projected
  line L29 (52.325, 47.25) -> (52.325, 48.5) projected
  line L30 (52.325, 48.5) -> (46, 48.5) projected
  line L31 (46, 48.5) -> (46, 51.5) projected
  line L32 (46, 51.5) -> (52.325, 51.5) projected
  line L33 (52.325, 51.5) -> (52.325, 52.75) projected
  line L34 (52.325, 52.75) -> (54.825, 52.75) projected
  line L35 (54.825, 52.75) -> (54.825, 51.5) projected
  line L36 (54.825, 51.5) -> (56.825, 51.5) projected
  line L37 (56.825, 51.5) -> (56.825, 55) projected
  line L38 (56.825, 55) -> (60, 55) projected
  line L39 (60, 55) -> (60, 65) projected
  line L40 (60, 65) -> (56.825, 65) projected
  line L41 (56.825, 65) -> (56.825, 75) projected
  line L42 (56.825, 75) -> (60, 75) projected
  line L43 (60, 75) -> (60, 86.825) projected
  line L44 (55, 86.825) -> (60, 86.825) projected
  line L45 (55, 90) -> (55, 86.825) projected
  line L46 (45, 90) -> (55, 90) projected
  line L47 (45, 86.825) -> (45, 90) projected
  line L48 (45, 86.825) -> (35, 86.825) projected
  line L49 (35, 90) -> (35, 86.825) projected
  line L50 (25, 90) -> (35, 90) projected
  line L51 (25, 86.825) -> (25, 90) projected
  line L52 (25, 86.825) -> (15, 86.825) projected
  line L53 (15, 90) -> (15, 86.825) projected
  line L54 (5, 90) -> (15, 90) projected
  line L55 (5, 86.825) -> (5, 90) projected
  line L56 (5, 86.825) -> (-5, 86.825) projected
  line L57 (-5, 90) -> (-5, 86.825) projected
  line L58 (-15, 90) -> (-5, 90) projected
  line L59 (-15, 86.825) -> (-15, 90) projected
  line L60 (-15, 86.825) -> (-25, 86.825) projected
  line L61 (-25, 90) -> (-25, 86.825) projected
  line L62 (-35, 90) -> (-25, 90) projected
  line L63 (-35, 86.825) -> (-35, 90) projected
  line L64 (-35, 86.825) -> (-45, 86.825) projected
  line L65 (-45, 90) -> (-45, 86.825) projected
  line L66 (-55, 90) -> (-45, 90) projected
  line L67 (-55, 86.825) -> (-55, 90) projected
  line L68 (-55, 86.825) -> (-60, 86.825) projected
  line L69 (-60, 75) -> (-60, 86.825) projected
  line L70 (-56.825, 75) -> (-60, 75) projected
  line L71 (-56.825, 75) -> (-56.825, 65) projected
  line L72 (-60, 65) -> (-56.825, 65) projected
  line L73 (-60, 55) -> (-60, 65) projected
  line L74 (-56.825, 55) -> (-60, 55) projected
  line L75 (-56.825, 55) -> (-56.825, 45) projected
  line L76 (-60, 45) -> (-56.825, 45) projected
  line L77 (-60, 35) -> (-60, 45) projected
  line L78 (-56.825, 35) -> (-60, 35) projected
  line L79 (-56.825, 35) -> (-56.825, 25) projected
  line L80 (-60, 25) -> (-56.825, 25) projected
  line L81 (-60, 15) -> (-60, 25) projected
  line L82 (-56.825, 15) -> (-60, 15) projected
  line L83 (-56.825, 15) -> (-56.825, 5) projected
  line L84 (-60, 5) -> (-56.825, 5) projected
  line L85 (-60, -5) -> (-60, 5) projected
  line L86 (-56.825, -5) -> (-60, -5) projected
  line L87 (-56.825, -5) -> (-56.825, -15) projected
  line L88 (-60, -15) -> (-56.825, -15) projected
  line L89 (-60, -25) -> (-60, -15) projected
  line L90 (-56.825, -25) -> (-60, -25) projected
  line L91 (-56.825, -25) -> (-56.825, -35) projected
  line L92 (-60, -35) -> (-56.825, -35) projected
  line L93 (-60, -45) -> (-60, -35) projected
  line L94 (-56.825, -45) -> (-60, -45) projected
  line L95 (-56.825, -45) -> (-56.825, -55) projected
  line L96 (-60, -55) -> (-56.825, -55) projected
  line L97 (-60, -65) -> (-60, -55) projected
  line L98 (-56.825, -65) -> (-60, -65) projected
  line L99 (-56.825, -65) -> (-56.825, -75) projected
  line L100 (-60, -75) -> (-56.825, -75) projected
  line L101 (-60, -75) -> (-60, -86.825) projected
  line L102 (-60, -86.825) -> (-55, -86.825) projected
  line L103 (-55, -86.825) -> (-55, -90) projected
  line L104 (-55, -90) -> (-45, -90) projected
  line L105 (-45, -90) -> (-45, -86.825) projected
  line L106 (-45, -86.825) -> (-35, -86.825) projected
  line L107 (-35, -86.825) -> (-35, -90) projected
  line L108 (-35, -90) -> (-25, -90) projected
  line L109 (-25, -90) -> (-25, -86.825) projected
  line L110 (-25, -86.825) -> (-15, -86.825) projected
  line L111 (-15, -86.825) -> (-15, -90) projected
  line L112 (-15, -90) -> (-5, -90) projected
  line L113 (-5, -90) -> (-5, -86.825) projected
  line L114 (-5, -86.825) -> (5, -86.825) projected
  line L115 (5, -86.825) -> (5, -90) projected
  line L116 (5, -90) -> (15, -90) projected
  line L117 (15, -90) -> (15, -86.825) projected
  line L118 (15, -86.825) -> (25, -86.825) projected
  line L119 (25, -86.825) -> (25, -90) projected
  line L120 (25, -90) -> (35, -90) projected
  line L121 (35, -90) -> (35, -86.825) projected
  line L122 (35, -86.825) -> (45, -86.825) projected
  line L123 (45, -86.825) -> (45, -90) projected
  line L124 (45, -90) -> (55, -90) projected
  line L125 (55, -90) -> (55, -86.825) projected
  line L126 (55, -86.825) -> (60, -86.825) projected
  line L127 (60, -86.825) -> (60, -75) projected
  line L128 (60, -75) -> (56.825, -75) projected
  line L129 (56.825, -75) -> (56.825, -65) projected
  line L130 (56.825, -65) -> (60, -65) projected
  line L131 (60, -65) -> (60, -55) projected
  line L132 (60, -55) -> (56.825, -55) projected
  line L133 (56.825, -55) -> (56.825, -51.5) projected
  line L134 (56.825, -51.5) -> (54.825, -51.5) projected
  line L135 (54.825, -51.5) -> (54.825, -52.75) projected
  line L136 (54.825, -52.75) -> (52.325, -52.75) projected
  line L137 (52.325, -52.75) -> (52.325, -51.5) projected
  line L138 (52.325, -51.5) -> (46, -51.5) projected
  line L139 (46, -51.5) -> (46, -48.5) projected
  line L140 (46, -48.5) -> (52.325, -48.5) projected
  line L141 (52.325, -48.5) -> (52.325, -47.25) projected
  line L142 (52.325, -47.25) -> (54.825, -47.25) projected
  line L143 (54.825, -47.25) -> (54.825, -48.5) projected
  circle A4 centre (22.9972, -27.4451) radius 3 projected
  circle A5 centre (-22.9972, 54) radius 3 projected
  circle A6 centre (22.9972, 27.4451) radius 3 projected
  circle A7 centre (-22.9972, -54) radius 3 projected
  circle A8 centre (-15, 8.175) radius 11 projected
  line L144 (-56.945, -34.88) -> (-56.945, -25.12)
  line L145 (-56.945, -25.12) -> (-60.12, -25.12)
  line L146 (-60.12, -25.12) -> (-60.12, -14.88)
  line L147 (-60.12, -14.88) -> (-56.945, -14.88)
  line L148 (-56.945, -14.88) -> (-56.945, -5.12)
  line L149 (-56.945, -5.12) -> (-60.12, -5.12)
  line L150 (-60.12, -5.12) -> (-60.12, 5.12)
  line L151 (-60.12, 5.12) -> (-56.945, 5.12)
  line L152 (-56.945, 5.12) -> (-56.945, 14.88)
  line L153 (-56.945, 14.88) -> (-60.12, 14.88)
  line L154 (-60.12, 14.88) -> (-60.12, 25.12)
  line L155 (-60.12, 25.12) -> (-56.945, 25.12)
  line L156 (-56.945, 25.12) -> (-56.945, 34.88)
  line L157 (-56.945, 34.88) -> (-60.12, 34.88)
  line L158 (-60.12, 34.88) -> (-60.12, 45.12)
  line L159 (-60.12, 45.12) -> (-56.945, 45.12)
  line L160 (-56.945, 45.12) -> (-56.945, 54.88)
  line L161 (-56.945, 54.88) -> (-60.12, 54.88)
  line L162 (-60.12, 54.88) -> (-60.12, 65.12)
  line L163 (-60.12, 65.12) -> (-56.945, 65.12)
  line L164 (-56.945, 65.12) -> (-56.945, 74.88)
  line L165 (-56.945, 74.88) -> (-60.12, 74.88)
  line L166 (-60.12, 74.88) -> (-60.12, 86.945)
  line L167 (-60.12, 86.945) -> (-55.12, 86.945)
  line L168 (-55.12, 86.945) -> (-55.12, 90.12)
  line L169 (-55.12, 90.12) -> (-44.88, 90.12)
  line L170 (-44.88, 90.12) -> (-44.88, 86.945)
  line L171 (-44.88, 86.945) -> (-35.12, 86.945)
  line L172 (-35.12, 86.945) -> (-35.12, 90.12)
  line L173 (-35.12, 90.12) -> (-24.88, 90.12)
  line L174 (-24.88, 90.12) -> (-24.88, 86.945)
  line L175 (-24.88, 86.945) -> (-15.12, 86.945)
  line L176 (-15.12, 86.945) -> (-15.12, 90.12)
  line L177 (-15.12, 90.12) -> (-4.88, 90.12)
  line L178 (-4.88, 90.12) -> (-4.88, 86.945)
  line L179 (-4.88, 86.945) -> (4.88, 86.945)
  line L180 (4.88, 86.945) -> (4.88, 90.12)
  line L181 (4.88, 90.12) -> (15.12, 90.12)
  line L182 (15.12, 90.12) -> (15.12, 86.945)
  line L183 (15.12, 86.945) -> (24.88, 86.945)
  line L184 (24.88, 86.945) -> (24.88, 90.12)
  line L185 (24.88, 90.12) -> (35.12, 90.12)
  line L186 (35.12, 90.12) -> (35.12, 86.945)
  line L187 (35.12, 86.945) -> (44.88, 86.945)
  line L188 (44.88, 86.945) -> (44.88, 90.12)
  line L189 (44.88, 90.12) -> (55.12, 90.12)
  line L190 (55.12, 90.12) -> (55.12, 86.945)
  line L191 (55.12, 86.945) -> (60.12, 86.945)
  line L192 (60.12, 86.945) -> (60.12, 74.88)
  line L193 (60.12, 74.88) -> (56.945, 74.88)
  line L194 (56.945, 74.88) -> (56.945, 65.12)
  line L195 (56.945, 65.12) -> (60.12, 65.12)
  line L196 (60.12, 65.12) -> (60.12, 54.88)
  line L197 (60.12, 54.88) -> (56.945, 54.88)
  line L198 (56.945, 54.88) -> (56.945, 51.38)
  line L199 (56.945, 51.38) -> (54.705, 51.38)
  line L200 (54.705, 51.38) -> (54.705, 52.63)
  line L201 (54.705, 52.63) -> (52.445, 52.63)
  line L202 (52.445, 52.63) -> (52.445, 51.38)
  line L203 (52.445, 51.38) -> (46.12, 51.38)
  line L204 (46.12, 51.38) -> (46.12, 48.62)
  line L205 (46.12, 48.62) -> (52.445, 48.62)
  line L206 (52.445, 48.62) -> (52.445, 47.37)
  line L207 (52.445, 47.37) -> (54.705, 47.37)
  line L208 (54.705, 47.37) -> (54.705, 48.62)
  line L209 (54.705, 48.62) -> (56.945, 48.62)
  line L210 (56.945, 48.62) -> (56.945, 45.12)
  line L211 (56.945, 45.12) -> (60.12, 45.12)
  line L212 (60.12, 45.12) -> (60.12, 34.88)
  line L213 (60.12, 34.88) -> (56.945, 34.88)
  line L214 (56.945, 34.88) -> (56.945, 25.12)
  line L215 (56.945, 25.12) -> (60.12, 25.12)
  line L216 (60.12, 25.12) -> (60.12, 14.88)
  line L217 (60.12, 14.88) -> (56.945, 14.88)
  line L218 (56.945, 14.88) -> (56.945, 5.12)
  line L219 (56.945, 5.12) -> (60.12, 5.12)
  line L220 (60.12, 5.12) -> (60.12, -5.12)
  line L221 (60.12, -5.12) -> (56.945, -5.12)
  line L222 (56.945, -5.12) -> (56.945, -14.88)
  line L223 (56.945, -14.88) -> (60.12, -14.88)
  line L224 (60.12, -14.88) -> (60.12, -25.12)
  line L225 (60.12, -25.12) -> (56.945, -25.12)
  line L226 (56.945, -25.12) -> (56.945, -34.88)
  line L227 (56.945, -34.88) -> (60.12, -34.88)
  line L228 (60.12, -34.88) -> (60.12, -45.12)
  line L229 (60.12, -45.12) -> (56.945, -45.12)
  line L230 (56.945, -45.12) -> (56.945, -48.62)
  line L231 (56.945, -48.62) -> (54.705, -48.62)
  line L232 (54.705, -48.62) -> (54.705, -47.37)
  line L233 (54.705, -47.37) -> (52.445, -47.37)
  line L234 (52.445, -47.37) -> (52.445, -48.62)
  line L235 (52.445, -48.62) -> (46.12, -48.62)
  line L236 (46.12, -48.62) -> (46.12, -51.38)
  line L237 (46.12, -51.38) -> (52.445, -51.38)
  line L238 (52.445, -51.38) -> (52.445, -52.63)
  line L239 (52.445, -52.63) -> (54.705, -52.63)
  line L240 (54.705, -52.63) -> (54.705, -51.38)
  line L241 (54.705, -51.38) -> (56.945, -51.38)
  line L242 (56.945, -51.38) -> (56.945, -54.88)
  line L243 (56.945, -54.88) -> (60.12, -54.88)
  line L244 (60.12, -54.88) -> (60.12, -65.12)
  line L245 (60.12, -65.12) -> (56.945, -65.12)
  line L246 (56.945, -65.12) -> (56.945, -74.88)
  line L247 (56.945, -74.88) -> (60.12, -74.88)
  line L248 (60.12, -74.88) -> (60.12, -86.945)
  line L249 (60.12, -86.945) -> (55.12, -86.945)
  line L250 (55.12, -86.945) -> (55.12, -90.12)
  line L251 (55.12, -90.12) -> (44.88, -90.12)
  line L252 (44.88, -90.12) -> (44.88, -86.945)
  line L253 (44.88, -86.945) -> (35.12, -86.945)
  line L254 (35.12, -86.945) -> (35.12, -90.12)
  line L255 (35.12, -90.12) -> (24.88, -90.12)
  line L256 (24.88, -90.12) -> (24.88, -86.945)
  line L257 (24.88, -86.945) -> (15.12, -86.945)
  line L258 (15.12, -86.945) -> (15.12, -90.12)
  line L259 (15.12, -90.12) -> (4.88, -90.12)
  line L260 (4.88, -90.12) -> (4.88, -86.945)
  line L261 (4.88, -86.945) -> (-4.88, -86.945)
  line L262 (-4.88, -86.945) -> (-4.88, -90.12)
  line L263 (-4.88, -90.12) -> (-15.12, -90.12)
  line L264 (-15.12, -90.12) -> (-15.12, -86.945)
  line L265 (-15.12, -86.945) -> (-24.88, -86.945)
  line L266 (-24.88, -86.945) -> (-24.88, -90.12)
  line L267 (-24.88, -90.12) -> (-35.12, -90.12)
  line L268 (-35.12, -90.12) -> (-35.12, -86.945)
  line L269 (-35.12, -86.945) -> (-44.88, -86.945)
  line L270 (-44.88, -86.945) -> (-44.88, -90.12)
  line L271 (-44.88, -90.12) -> (-55.12, -90.12)
  line L272 (-55.12, -90.12) -> (-55.12, -86.945)
  line L273 (-55.12, -86.945) -> (-60.12, -86.945)
  line L274 (-60.12, -86.945) -> (-60.12, -74.88)
  line L275 (-60.12, -74.88) -> (-56.945, -74.88)
  line L276 (-56.945, -74.88) -> (-56.945, -65.12)
  line L277 (-56.945, -65.12) -> (-60.12, -65.12)
  line L278 (-60.12, -65.12) -> (-60.12, -54.88)
  line L279 (-60.12, -54.88) -> (-56.945, -54.88)
  line L280 (-56.945, -54.88) -> (-56.945, -45.12)
  line L281 (-56.945, -45.12) -> (-60.12, -45.12)
  line L282 (-60.12, -45.12) -> (-60.12, -34.88)
  line L283 (-60.12, -34.88) -> (-56.945, -34.88)
  circle A9 centre (-22.9972, -54) radius 2.88
  circle A10 centre (22.9972, -27.4451) radius 2.88
  circle A11 centre (-15, 8.175) radius 10.88
  circle A12 centre (22.9972, 27.4451) radius 2.88
  circle A13 centre (38.1, 0) radius 0.958
  circle A14 centre (45.72, 0) radius 0.958
  line L284 (43.695, -13.215) -> (40.125, -13.215)
  line L285 (40.125, -13.215) -> (40.125, -2.025)
  line L286 (40.125, -2.025) -> (43.695, -2.025)
  line L287 (43.695, -2.025) -> (43.695, -13.215)
  circle A15 centre (45.72, -15.24) radius 0.958
  circle A16 centre (38.1, -15.24) radius 0.958
  circle A17 centre (-22.9972, 54) radius 2.88
  point P0 (-361.08, 0)
  dimension "d54" = 0.12
  dimension "d55" = 0.12
  dimension "d56" = 0.12
  dimension "d57" = 0.12
  dimension "d58" = 0.12
  dimension "d59" = 0.12
  dimension "d60" = 0.12
  dimension "d61" = 0.12
  dimension "d62" = 0.12
  dimension "d63" = 0.12
  dimension "d64" = 0.12
  constraints: 288 end point, 9 centre point, 142 other
  measures "d54" distance between parallel lines of L91 L144
  measures "d55" radial gap between concentric circles of A7 A9
  measures "d56" radial gap between concentric circles of A4 A10
  measures "d57" radial gap between concentric circles of A8 A11
  measures "d58" radial gap between concentric circles of A6 A12
  measures "d59" radial gap between concentric circles of A3 A13
  measures "d60" radial gap between concentric circles of A1 A14
  measures "d61" distance between parallel lines of L3 L287
  measures "d62" radial gap between concentric circles of A2 A15
  measures "d63" radial gap between concentric circles of A0 A16
  measures "d64" radial gap between concentric circles of A5 A17
extrude "Extrusion3" add sketch "Sketch3" along normal blind 3.175 contours L0 L1 L2 L3 | A0 | A1 | A2 | A3 | L143 L142 L141 L140 L139 L138 L137 L136 L135 L134 L133 L132 L131 L130 L129 L128 L127 L126 L125 L124 L123 L122 L121 L120 L119 L118 L117 L116 L115 L114 L113 L112 L111 L110 L109 L108 L107 L106 L105 L104 L103 L102 L101 L100 L99 L98 L97 L96 L95 L94 L93 L92 L91 L90 L89 L88 L87 L86 L85 L84 L83 L82 L81 L80 L79 L78 L77 L76 L75 L74 L73 L72 L71 L70 L69 L68 L67 L66 L65 L64 L63 L62 L61 L60 L59 L58 L57 L56 L55 L54 L53 L52 L51 L50 L49 L48 L47 L46 L45 L44 L43 L42 L41 L40 L39 L38 L37 L36 L35 L34 L33 L32 L31 L30 L29 L28 L27 L26 L25 L24 L23 L22 L21 L20 L19 L18 L17 L16 L15 L14 L13 L12 L11 L10 L9 L8 L7 L6 L5 L4 | A4 | A5 | A6 | A7 | A8 | L144 L145 L146 L147 L148 L149 L150 L151 L152 L153 L154 L155 L156 L157 L158 L159 L160 L161 L162 L163 L164 L165 L166 L167 L168 L169 L170 L171 L172 L173 L174 L175 L176 L177 L178 L179 L180 L181 L182 L183 L184 L185 L186 L187 L188 L189 L190 L191 L192 L193 L194 L195 L196 L197 L198 L199 L200 L201 L202 L203 L204 L205 L206 L207 L208 L209 L210 L211 L212 L213 L214 L215 L216 L217 L218 L219 L220 L221 L222 L223 L224 L225 L226 L227 L228 L229 L230 L231 L232 L233 L234 L235 L236 L237 L238 L239 L240 L241 L242 L243 L244 L245 L246 L247 L248 L249 L250 L251 L252 L253 L254 L255 L256 L257 L258 L259 L260 L261 L262 L263 L264 L265 L266 L267 L268 L269 L270 L271 L272 L273 L274 L275 L276 L277 L278 L279 L280 L281 L282 L283
equation "\"d0\" = laserKerf"
equation "\"d1\" = laserKerf"
equation "\"d2\" = laserKerf"
equation "\"d3\" = laserKerf"
equation "\"d4\" = laserKerf"
equation "\"d5\" = laserKerf"
equation "\"d6\" = laserKerf"
equation "\"d7\" = laserKerf"
equation "\"d8\" = laserKerf"
equation "\"d9\" = laserKerf"
equation "\"d10\" = laserKerf"
equation "\"d11\" = laserKerf"
equation "\"d12\" = laserKerf"
equation "\"d13\" = laserKerf"
equation "\"d14\" = laserKerf"
equation "\"d15\" = laserKerf"
equation "\"d16\" = laserKerf"
equation "\"d17\" = laserKerf"
equation "\"d18\" = laserKerf"
equation "\"d19\" = laserKerf"
equation "\"d20\" = laserKerf"
equation "\"d21\" = laserKerf"
equation "\"d22\" = laserKerf"
equation "\"d23\" = laserKerf"
equation "\"d24\" = laserKerf"
equation "\"d25\" = laserKerf"
equation "\"d26\" = laserKerf"
equation "\"d27\" = laserKerf"
equation "\"d28\" = laserKerf"
equation "\"d29\" = laserKerf"
equation "\"d30\" = laserKerf"
equation "\"d31\" = laserKerf"
equation "\"d32\" = laserKerf"
equation "\"d33\" = laserKerf"
equation "\"d34\" = laserKerf"
equation "\"d35\" = laserKerf"
equation "\"d36\" = laserKerf"
equation "\"d37\" = laserKerf"
equation "\"d38\" = laserKerf"
equation "\"d39\" = materialThickness"
equation "\"materialThickness\" = 3.175"
equation "\"laserKerf\" = 0.12"
equation "\"cardPinDiameter\" = 3"
equation "\"centeralShaftDiameter\" = 8"
equation "\"cardWidth\" = 85.6"
equation "\"cardHeight\" = 53.98"
equation "\"cardThickness\" = 0.76"
equation "\"cardFillet\" = 2.88"
equation "\"cardClearence\" = 0.5"
equation "\"bearingOd\" = 22"
equation "\"bearingWidth\" = 8"
equation "\"axleHeight\" = 95"
equation "\"nutTrapClearence\" = 2"
equation "\"nutTrapwidth\" = 5.5"
equation "\"nutTrapDepth\" = 2.5"
equation "\"magnetDiameter\" = 6"
equation "\"magnetLength\" = 3"
equation "\"magnetProtusion\" = 0.25"
equation "\"spoolThickness\" = 5.588"
body "Solid1"
